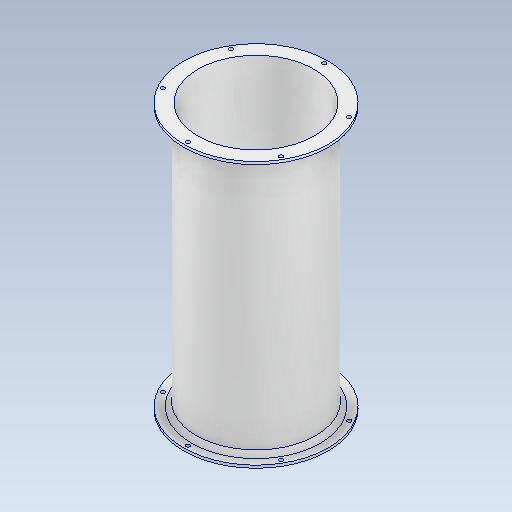
# Autodesk Inventor part: Link_3
Saved by Autodesk Inventor 2021 (Build 250183000, 183)
## iProperties
Created: 2020-05-10
Part Number: Link_3
Material: Aluminum 6061
Document SubType Name: Modeling
Designer: avi41
Density: 2.7 g/cm^3
Appearance: Aluminum - Flat
Author: avi41
Autodesk Inventor part; units mm, degrees
ref_plane "YZ Plane" through (0, 0, 0) normal (1, 0, 0) x (0, 1, 0)
ref_plane "XZ Plane" through (0, 0, 0) normal (0, 1, 0) x (-1, 0, 0)
ref_plane "XY Plane" through (0, 0, 0) normal (0, 0, 1) x (1, 0, 0)
sketch "Sketch1" plane through (0, 0, 0) normal (0, 0, 1) x (1, 0, 0)
  line L0 (-16.3, 0) -> (97.8, 0) construction
  line L1 (0, 210) -> (0, -210) construction
  line L2 (65.5, -150) -> (65.5, 150)
  line L3 (65.5, 150) -> (67.5, 150)
  line L4 (81.5, -147) -> (81.5, -150)
  line L5 (81.5, -150) -> (65.5, -150)
  line L6 (67.5, -142) -> (67.5, 142)
  line L7 (81.5, -147) -> (72.5, -147)
  line L8 (72.5, -147) -> (67.5, -142)
  line L9 (81.5, 150) -> (65.5, 150)
  line L10 (81.5, 150) -> (81.5, 147)
  line L11 (81.5, 147) -> (72.5, 147)
  line L12 (72.5, 147) -> (67.5, 142)
  point P0 (0, 0)
  dimension "d0" = 300
  dimension "d5" = 81.5
  dimension "d6" = 2
  dimension "d7" = 9
  dimension "d8" = 5
  dimension "d9" = 45
  dimension "d10" = 16
  dimension "d11" = 3
  dimension "d12" = 3
  dimension "d13" = 9
  dimension "d14" = 45
  dimension "d15" = 5
  constraints: 22 end point, 4 perpendicular, 3 horizontal, 2 vertical, 1 other
  measures "d0" distance of L2.start L2.end
  measures "d5" distance between parallel lines of L1 L4
  measures "d6" distance between parallel lines of L2 L6
  measures "d7" distance of L4.start L7.end
  measures "d8" horizontal distance of L7.end L6.start
  measures "d9" angle of L5 L8
  measures "d10" distance of L4.end L2.start
  measures "d11" distance between parallel lines of L5 L7
  measures "d12" distance of L9.start L10.end
  measures "d13" distance of L10.end L11.end
  measures "d14" angle of L6 L12
  measures "d15" horizontal distance of L6.end L11.end
revolve "Revolution1" add sketch "Sketch1" angle 360 about axis through (0, 0, 0) along (0, -1, 0)
sketch "Sketch2" plane through (0, -150, 0) normal (0, -1, 0) x (1, 0, 0)
  line L0 (0, 114.1) -> (0, -114.1) construction
  line L1 (-114.1, 0) -> (114.1, 0) construction
  circle A0 centre (0, 0) radius 81.5 construction
  circle A1 centre (0, 0) radius 65.5 construction
  circle A2 centre (0, 0) radius 77 construction
  circle A3 centre (0, 0) radius 72.5 construction
  point P0 (0, 77)
  point P1 (-66.684, 38.5)
  point P2 (-66.684, -38.5)
  point P3 (0, -77)
  point P4 (66.684, -38.5)
  point P5 (66.684, 38.5)
  dimension "d16" = 4.5
  dimension "d20" = 360
  dimension "d29" = 4.5
  constraints: 1 coincident, 1 point on line, 1 vertical alignment, 9 other
hole "Hole1" at (0, -150, 77) at (-66.684, -150, 38.5) at (-66.684, -150, -38.5) at (0, -150, -77) at (66.684, -150, -38.5) at (66.684, -150, 38.5) direction (0, 1, 0) diameter 4.5 depth 13 tip angle 118 clearance for "Flat Head Machine Screw" size "M4" standard "Ansi Metric M Profile"
mirror "Mirror1" about plane through (0, 0, 0) normal (0, 1, 0) of "Hole1"
equation "\"d16\" = d29"
equation "\"d12\" = d11"
equation "\"d13\" = d7"
equation "\"d14\" = d9"
equation "\"d15\" = d8"
body "Solid1"
